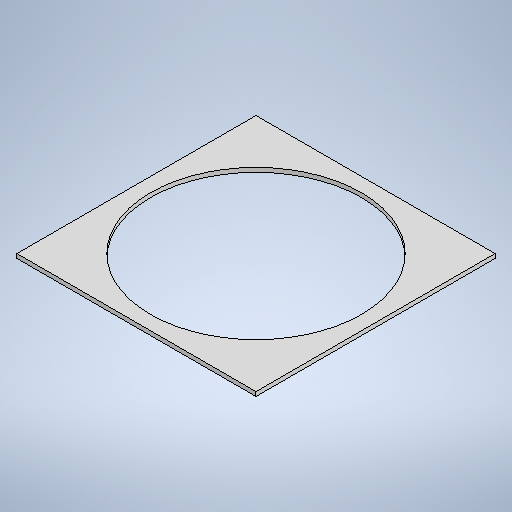
# Autodesk Inventor part: drain bottom plate
Saved by Autodesk Inventor 2025 (Build 290162010, 162A)
## iProperties
Created: 2024-12-09
Part Number: drain bottom plate
Material: Stainless Steel
Document SubType Name: Sheet Metal
Designer: user
Mass: 269.485 g
Surface Area: 259.108 cm^2
Volume: 33.6856 cm^3
Density: 8 g/cm^3
Sheet Metal Rule: AISI304 3mm Die 32
Sheet Metal Width: 170,000 mm
Sheet Metal Length: 170,000 mm
Sheet Metal Area: 28900,000 mm^2
Appearance: Default
Flat Pattern Width: 17 cm
Flat Pattern Length: 17 cm
Flat Pattern Area: 289 cm^2
Author: user
Autodesk Inventor part; units mm, degrees
ref_plane "YZ Plane" through (0, 0, 0) normal (1, 0, 0) x (0, 1, 0)
ref_plane "XZ Plane" through (0, 0, 0) normal (0, 1, 0) x (-1, 0, 0)
ref_plane "XY Plane" through (0, 0, 0) normal (0, 0, 1) x (1, 0, 0)
sketch "Sketch1" plane through (0, 0, 0) normal (0, 0, 1) x (1, 0, 0)
  line L0 (-85, -85) -> (85, -85)
  line L1 (85, -85) -> (85, 85)
  line L2 (85, 85) -> (-85, 85)
  line L3 (-85, 85) -> (-85, -85)
  line L4 (-85, -85) -> (85, 85) construction
  line L5 (85, -85) -> (-85, 85) construction
  circle A0 centre (0, 0) radius 75
  dimension "d0" = 170
  dimension "d1" = 170
  dimension "d22" = 150
  measures "d0" distance of L2.end L1.end
  measures "d1" distance of L1.end L0.end
  measures "d22" diameter of A0
extrude "Plate1" add sketch "Sketch1" along normal blind 3
equation "\"d1\" = d0"
equation "\"d2\" = Thickness"
equation "\"BendReliefWidth\" = Thickness"
equation "\"BendReliefDepth\" = 0.5 * Thickness"
equation "\"CornerReliefSize\" = 4 * Thickness"
equation "\"MinimumRemnant\" = 2 * Thickness"
equation "\"TransitionRadius\" = BendRadius"
equation "\"JacobiRadiusSize\" = BendRadius"
equation "\"GapSize\" = Thickness"
equation "\"Thickness\" = 3"
equation "\"BendRadius\" = 5"
body "Solid1"
